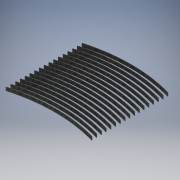
# Autodesk Inventor part: bent slat
Saved by Autodesk Inventor 2019 (Build 230136000, 136)
## iProperties
Created: 2018-08-04
Part Number: bent slat
Material: Steel
Document SubType Name: Modeling
Designer: torba
Density: 7.85 g/cm^3
Appearance: Plate
Author: torba
Autodesk Inventor part; units mm, degrees
ref_plane "YZ Plane" through (0, 0, 0) normal (1, 0, 0) x (0, 1, 0)
ref_plane "XZ Plane" through (0, 0, 0) normal (0, 1, 0) x (-1, 0, 0)
ref_plane "XY Plane" through (0, 0, 0) normal (0, 0, 1) x (1, 0, 0)
sketch "Sketch1" plane through (0, 0, 0) normal (0, 1, 0) x (-1, 0, 0)
  line L0 (73.025, 76.2127) -> (73.025, -1282.6873)
  line L1 (0, -4.7625) -> (-3.175, -4.7625)
  line L2 (-3.175, 0) -> (0, 0)
  line L3 (-3.175, -4.7625) -> (-3.175, 0)
  line L4 (3.175, 0) -> (3.175, -4.7625)
  line L5 (0, -4.7625) -> (3.175, -4.7625)
  line L6 (3.175, 0) -> (0, 0)
  line L7 (-603.2248, -75.0951) -> (-603.2248, -79.8576)
  line L8 (-609.6, -79.8576) -> (-606.3998, -79.8576)
  line L9 (-603.2248, -79.8576) -> (-606.3998, -79.8576)
  line L10 (-606.425, -75.0951) -> (-603.2248, -75.0951)
  line L11 (-606.425, -75.0951) -> (-609.6, -75.0951)
  line L12 (-609.6, -79.8576) -> (-609.6, -75.0951)
  line L13 (-1209.675, 0.0127) -> (-1209.675, 0)
  line L14 (-1216.025, -3.9489) -> (-1216.025, -3.9002)
  line L15 (-1285.875, 14.791) -> (-1285.875, 20.0374)
  arc A0 (-1212.85, 0.0127) -> (0, 0) centre (-606.3998, 2410.819) ccw
  arc A1 (-1212.85, -4.7498) -> (0, -4.7625) centre (-606.3998, 2406.0565) ccw
  line L16 (0, 0) -> (73.025, 20.0374)
  line L17 (0, -4.7625) -> (73.025, 14.791)
  line L18 (-1212.85, 0.0127) -> (-1285.875, 20.0374)
  line L19 (-1212.85, -4.7498) -> (-1285.875, 14.791)
  constraints: 40 end point, 10 parallel, 6 point on circle, 4 point on line, 3 tangent, 2 centre point, 1 equal radius, 1 horizontal, 1 vertical
extrude "Extrusion1" add sketch "Sketch1" along normal blind 50.8 contours L0 L17 L4 L6 L16 | A0 L3 L2 | L6 L4 L17 L1 L3 A0 | L3 L1 A1 L7 L10 A0 | L10 L7 A1 L12 L11 | L11 L12 A1 L19 L15 L18 A0
pattern_linear "Rectangular Pattern1" count 17 spacing 75.1078 along (0, 0, -1) of "Extrusion1"
body "Solid1"
